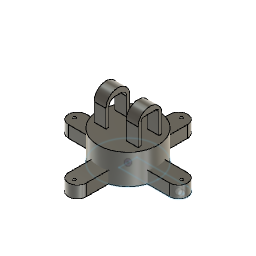
Base 2 v4 (Autodesk Fusion 360 design; units mm, degrees)
Autodesk Fusion 360 part; units mm, degrees
note: some values were not read from the file. Chosen so that the rebuilt part matches the saved one: that a step has no effect. Set by a fixed rule: which sketch regions a step uses.
sketch "Sketch1" plane through (0, 0, 0) normal (0, 0, 1) x (1, 0, 0)
  circle A0 centre (0, 0) radius 50
  constraint coincident A0.centre origin
extrude "Extrude1" add sketch "Sketch1" along normal blind 50 makes body 1
sketch "Sketch2" plane through (0, 0, 0) normal (0, 0, 1) x (1, 0, 0)
  line L0 (0, -15) -> (85, -15)
  line L1 (85, 15) -> (0, 15)
  line L2 (0, 15) -> (0, -15)
  arc A0 (85, -15) -> (85, 15) centre (85, 0) ccw
  constraint horizontal L0
  constraint perpendicular L0 L2
extrude "Extrude2" add sketch "Sketch2" along normal blind 20 separate body makes body 2
pattern_circular "C-Pattern2" [no effect]
sketch "Sketch6" plane through (0, 0, 0) normal (0, 0, 1) x (1, 0, 0)
  circle A0 centre (90, 0) radius 2.5
  dimension "d11" = 5
  measures "d11" diameter of A0
extrude "Extrude4" cut sketch "Sketch6" along normal through all bodies 2
pattern_circular "C-Pattern3" count 4 over 360 about axis through (0, 0, 1.75) along (0, 0, 1) of bodies 2 makes body 3 at (0, 29.1667, 0) makes body 4 at (-29.1667, 0, 0) makes body 5 at (0, -29.1667, 0)
sketch "Sketch13" plane through (0, 0, 50) normal (0, 0, 1) x (-1, 0, 0)
  circle A0 centre (0, 0) radius 50
sketch "Sketch15" plane through (-15, 0, 0) normal (-1, 0, 0) x (0, -1, 0)
  line L0 (-40, 50) -> (40, 50)
  line L1 (40, 50) -> (40, 100)
  line L2 (40, 100) -> (-40, 100)
  line L3 (-40, 100) -> (-40, 50)
  line L4 (-20, 50) -> (20, 50)
  line L5 (20, 50) -> (20, 80)
  line L6 (-20, 80) -> (-20, 50)
  arc A0 (20, 80) -> (-20, 80) centre (0, 80) ccw
  constraint horizontal L4
  constraint vertical L5
  constraint vertical L6
  constraint coincident L0 L4.start
extrude "Extrude12" add sketch "Sketch15" along normal blind 20 from surface at 2 contours L0 L4 L5 L6 A0 bodies 1
extrude "Extrude13" [no effect]
sketch "Sketch17" plane through (-37, 0, 0) normal (-1, 0, 0) x (0, -1, 0)
  arc A0 (20, 80) -> (-20, 80) centre (0, 80) ccw
  line L0 (-20, 80) -> (-20, 50)
  line L1 (-20, 50) -> (20, 50)
  line L2 (20, 50) -> (20, 80)
  line L3 (-5, 90) -> (5, 90)
  line L4 (15, 80) -> (15, 50)
  line L5 (15, 50) -> (-15, 50)
  line L6 (-15, 50) -> (-15, 80)
  arc A1 (-5, 90) -> (-15, 80) centre (-5, 80) ccw
  arc A2 (15, 80) -> (5, 90) centre (5, 80) ccw
  point P0 (-15, 90)
  point P1 (15, 90)
  dimension "d48" = 30
  dimension "d49" = 40
  dimension "d50" = 5
  dimension "d51" = 10
  constraint horizontal L3
  constraint vertical L4
  constraint horizontal L5
  constraint vertical L6
  constraint coincident L1 L4.end
  constraint coincident P0 L3
  constraint coincident P0 L6
  constraint tangent L3 A1
  constraint tangent L6 A1
  constraint coincident P1 L3
  constraint coincident P1 L4
  constraint tangent L3 A2
  constraint tangent L4 A2
  constraint equal A1 A2
  measures "d48" distance of P0 P1
  measures "d49" distance of P0 L5.end
  measures "d50" distance of L0 L6
  measures "d51" radius of A1
extrude "Extrude14" cut sketch "Sketch17" against normal blind 20 contours L1 L3 L4 L5 L6 A1 A2 bodies 1
pattern_circular "C-Pattern5" count 2 over 360 about axis through (0, 0, 1.75) along (0, 0, 1) of "Extrude12"
sketch "Sketch18" plane through (37, 0, 0) normal (1, 0, 0) x (0, 1, 0)
  arc A0 (20, 80) -> (-20, 80) centre (0, 80) ccw
  line L0 (-20, 80) -> (-20, 50)
  line L1 (-20, 50) -> (20, 50)
  line L2 (20, 50) -> (20, 80)
  line L3 (-10, 90) -> (10, 90)
  line L4 (15, 85) -> (15, 50)
  line L5 (15, 50) -> (-15, 50)
  line L6 (-15, 50) -> (-15, 85)
  arc A1 (-10, 90) -> (-15, 85) centre (-10, 85) ccw
  arc A2 (15, 85) -> (10, 90) centre (10, 85) ccw
  point P0 (-15, 90)
  point P1 (15, 90)
  dimension "d56" = 30
  dimension "d57" = 5
  dimension "d58" = 5
  constraint horizontal L3
  constraint vertical L4
  constraint horizontal L5
  constraint vertical L6
  constraint coincident L1 L4.end
  constraint coincident P0 L3
  constraint coincident P0 L6
  constraint tangent L3 A1
  constraint tangent L6 A1
  constraint coincident P1 L3
  constraint coincident P1 L4
  constraint tangent L3 A2
  constraint tangent L4 A2
  constraint equal A1 A2
  measures "d56" distance of P0 P1
  measures "d57" distance of L0 L6
  measures "d58" radius of A1
extrude "Extrude15" cut sketch "Sketch18" against normal blind 20 contours L1 L3 L4 L5 L6 A1 A2 bodies 1
sketch "Sketch19" plane through (0, 0, 0) normal (0, 0, 1) x (1, 0, 0)
  circle A0 centre (0, 0) radius 40
  constraint coincident A0.centre origin
extrude "Extrude16" cut sketch "Sketch19" along normal blind 40 bodies 1 2 3 4 5
sketch "Sketch20" plane through (0, 0, 0) normal (0, 0, 1) x (1, 0, 0)
